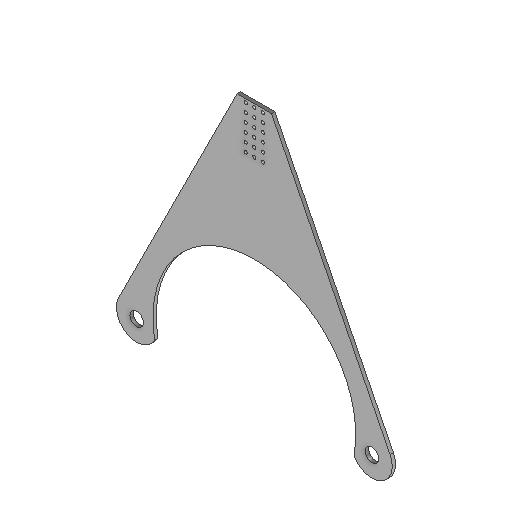
# Autodesk Inventor part: Chapa Base - Hand
Saved by Autodesk Inventor 2025.3 (Build 293356000, 356)
## iProperties
Created: 2026-05-13
Part Number: Chapa Base - Hand
Material: Genérico
Document SubType Name: Modeling
Designer: djair.oliveira
Density: 1 g/cm^3
Appearance: Padrão
Author: djair.oliveira
Autodesk Inventor part; units mm, degrees
ref_plane "YZ Plane" through (0, 0, 0) normal (1, 0, 0) x (0, 1, 0)
ref_plane "XZ Plane" through (0, 0, 0) normal (0, 1, 0) x (-1, 0, 0)
ref_plane "XY Plane" through (0, 0, 0) normal (0, 0, 1) x (1, 0, 0)
sketch "Esboço1" plane through (0, 0, 0) normal (0, 0, 1) x (1, 0, 0)
  line L0 (25.4, -75) -> (-25.4, -75)
  line L1 (-25.4, -75) -> (-25.4, 75)
  line L2 (-25.4, 75) -> (25.4, 75)
  line L3 (25.4, 75) -> (25.4, -75)
  line L4 (25.4, -75) -> (-25.4, 75) construction
  line L5 (-25.4, -75) -> (25.4, 75) construction
  circle A0 centre (0, -274.187) radius 150
  circle A1 centre (0, -274.187) radius 200.8
  line L6 (-25.4, 75) -> (-200.8, -274.187)
  line L7 (0, -274.187) -> (0, 0)
  line L8 (25.4, -75) -> (-25.4, 75) construction
  line L9 (25.4, 75) -> (200.8, -274.187)
  circle A2 centre (-173.992, -287.653) radius 30
  circle A3 centre (173.992, -287.653) radius 30
  circle A4 centre (-173.992, -287.653) radius 10
  circle A5 centre (173.992, -287.653) radius 10
  circle A6 centre (0, 70) radius 2.5
  circle A7 centre (12.7, 70) radius 2.5
  circle A8 centre (-12.7, 70) radius 2.5
  circle A9 centre (0, 57.3) radius 2.5
  circle A10 centre (12.7, 57.3) radius 2.5
  circle A11 centre (-12.7, 57.3) radius 2.5
  circle A12 centre (0, 44.6) radius 2.5
  circle A13 centre (12.7, 44.6) radius 2.5
  circle A14 centre (-12.7, 44.6) radius 2.5
  circle A15 centre (0, 31.9) radius 2.5
  circle A16 centre (12.7, 31.9) radius 2.5
  circle A17 centre (-12.7, 31.9) radius 2.5
  circle A18 centre (0, 19.2) radius 2.5
  circle A19 centre (12.7, 19.2) radius 2.5
  circle A20 centre (-12.7, 19.2) radius 2.5
  circle A21 centre (0, 6.5) radius 2.5
  circle A22 centre (12.7, 6.5) radius 2.5
  circle A23 centre (-12.7, 6.5) radius 2.5
  point P0 (-147.4627, -301.6599)
  point P1 (147.4627, -301.6599)
  dimension "d5" = 60
  dimension "d0" = 50.8
  dimension "d1" = 300
  dimension "d3" = 150
  dimension "d4" = 50.8
  dimension "d6" = 20
  dimension "d7" = 20
  dimension "d8" = 5
  dimension "d9" = 5
  dimension "d12" = 12.7
  dimension "d15" = 12.7
  constraints: 23 centre point, 20 end point, 4 symmetric about line, 3 coincident, 3 parallel, 2 horizontal, 2 midpoint, 2 point on circle, 1 perpendicular, 1 vertical, 1 vertical alignment, 38 other
  measures "d0" distance of L1.end L2.end
  measures "d1" diameter of A0
  measures "d3" distance of L0.end L1.end
  measures "d4" radial gap between concentric circles of A1 A0
  measures "d6" diameter of A4
  measures "d7" diameter of A5
  measures "d8" diameter of A6
  measures "d9" distance from line of L2 A6.centre
  measures "d12" distance of A6.centre A7.centre
  measures "d15" distance of A6.centre A9.centre
extrude "Extrusão1" add sketch "Esboço1" along normal blind 5 contours A1 L9 A3 A0 L7 L0 | A1 L1 L2 L3 | L3 L9 A1 | L0 L7 A1 | L7 A0 A2 L6 A1 L0 | L0 A1 L7 | A1 L6 L1 | A3 A1 | A1 A3 A0 | A0 A2 A1 | A1 A2
